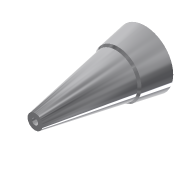
# Autodesk Inventor part: PP-02
Saved by Autodesk Inventor 2022 (Build 260148000, 148)
## iProperties
Created: 2008-09-23
Part Number: PP-02
Document SubType Name: Modeling
Designer: Mark Flayler
Mass: 1.76892 g
Surface Area: 4.74406 cm^2
Volume: 0.225054 cm^3
Density: 7.86 g/cm^3
Material: Steel, Mild
Description: CONE
Appearance: Aluminum - Polished
Author: Mark Flayler
Autodesk Inventor part; units mm, degrees
ref_plane "YZ Plane" through (0, 0, 0) normal (1, 0, 0) x (0, 1, 0)
ref_plane "XZ Plane" through (0, 0, 0) normal (0, 1, 0) x (-1, 0, 0)
ref_plane "XY Plane" through (0, 0, 0) normal (0, 0, 1) x (1, 0, 0)
sketch "Sketch1" plane through (0, 0, 0) normal (0, 0, 1) x (1, 0, 0)
  line L0 (0, 0) -> (0, 16.2)
  line L1 (0.45, 0) -> (1.1, 0)
  line L2 (1.1, 0) -> (3.1983, 11.9)
  line L3 (3.1983, 11.9) -> (3.4623, 12.2146)
  line L4 (3.4623, 12.2146) -> (4.165, 16.2)
  line L5 (4.165, 16.2) -> (2.59, 16.2)
  line L6 (2.59, 16.2) -> (2.59, 11.05)
  line L7 (2.59, 11.05) -> (1.7521, 11.05)
  line L8 (1.7521, 11.05) -> (1.7521, 8.2)
  line L9 (1.7521, 8.2) -> (1.4, 6.3)
  line L10 (1.4, 6.3) -> (0.45, 6.3)
  line L11 (0.45, 6.3) -> (0.45, 0)
  dimension "d0" = 30
  dimension "d1" = 100.5
  dimension "d2" = 0.9
  dimension "d3" = 2.2
  dimension "d4" = 6.3
  dimension "d5" = 16.2
  dimension "d6" = 8.2
  dimension "d7" = 11.05
  dimension "d8" = 2.8
  dimension "d9" = 5.18
  dimension "d10" = 11.9
  dimension "d11" = 8.33
  dimension "d12" = 80
  constraints: 24 end point, 6 perpendicular, 2 horizontal alignment, 2 parallel, 1 vertical
  measures "d0" angle of L2 L3
  measures "d1" angle of L1 L9
  measures "d2" diameter of L11 L0
  measures "d3" diameter of L1.end L0
  measures "d4" distance from line of L0.start L10
  measures "d5" distance from line of L0.start L5
  measures "d6" vertical distance of L0.start L8.end
  measures "d7" vertical distance of L0.start L7.end
  measures "d8" diameter of L9.end L0
  measures "d9" diameter of L5.end L0
  measures "d10" vertical distance of L0.start L2.end
  measures "d11" diameter of L4.end L0
  measures "d12" angle of L1 L2
revolve "Revolution1" add sketch "Sketch1" angle 360 about axis through (0, 0, 0) along (0, 1, 0)
body "Solid1"
